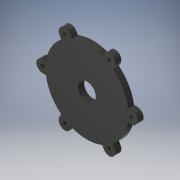
# Autodesk Inventor part: TA01
Saved by Autodesk Inventor 2017 (Build 210142000, 142)
## iProperties
Created: 2018-10-09
Part Number: TA01
Material: ABS Plastic
Document SubType Name: Modeling
Designer: Zach
Density: 1.06 g/cm^3
Appearance: Smooth - Black
Author: Zach
Autodesk Inventor part; units mm, degrees
ref_plane "YZ Plane" through (0, 0, 0) normal (1, 0, 0) x (0, 1, 0)
ref_plane "XZ Plane" through (0, 0, 0) normal (0, 1, 0) x (-1, 0, 0)
ref_plane "XY Plane" through (0, 0, 0) normal (0, 0, 1) x (1, 0, 0)
sketch "Sketch1" plane through (0, 0, 0) normal (0, 0, 1) x (1, 0, 0)
  circle A0 centre (0, 0) radius 15
  circle A1 centre (0, 0) radius 68.75
  circle A2 centre (-50, 0) radius 3
  circle A3 centre (-25, -43.3013) radius 3
  circle A4 centre (25, -43.3013) radius 3
  circle A5 centre (50, 0) radius 3
  circle A6 centre (25, 43.3013) radius 3
  circle A7 centre (-25, 43.3013) radius 3
  dimension "d0" = 30
  dimension "d1" = 137.5
  dimension "d2" = 6
  dimension "d6" = 360
  dimension "d15" = 50
  constraints: 8 centre point, 2 coincident, 1 horizontal alignment, 13 other
  measures "d0" diameter of A0
  measures "d1" diameter of A1
  measures "d2" diameter of A2
  measures "d15" distance of point (0, 0) A2.centre
extrude "Extrusion1" add sketch "Sketch1" along normal blind 10 contours A1 | A2 | A3 | A4 | A5 | A6 | A7
sketch "Sketch5" plane through (0, 0, 0) normal (0, 0, -1) x (-1, 0, 0)
  circle A0 centre (74, 0) radius 10
  line L0 (74, 10) -> (68.0188, 10)
  line L1 (74, -10) -> (68.0188, -10)
  line L2 (68.0188, 10) -> (68.0188, -10)
  circle A1 centre (74, 0) radius 3
  circle A2 centre (0, 0) radius 68.75 construction
  line L3 (74, 0) -> (0, 0) construction
  circle A3 centre (50.5575, 0) radius 3 construction
  circle A4 centre (37, 64.0859) radius 10
  line L4 (28.3397, 69.0859) -> (25.3492, 63.906)
  line L5 (45.6603, 59.0859) -> (42.6697, 53.906)
  line L6 (25.3492, 63.906) -> (42.6697, 53.906)
  circle A5 centre (37, 64.0859) radius 3
  circle A6 centre (-37, 64.0859) radius 10
  line L7 (-45.6603, 59.0859) -> (-42.6697, 53.906)
  line L8 (-28.3397, 69.0859) -> (-25.3492, 63.906)
  line L9 (-42.6697, 53.906) -> (-25.3492, 63.906)
  circle A7 centre (-37, 64.0859) radius 3
  circle A8 centre (-74, 0) radius 10
  line L10 (-74, -10) -> (-68.0188, -10)
  line L11 (-74, 10) -> (-68.0188, 10)
  line L12 (-68.0188, -10) -> (-68.0188, 10)
  circle A9 centre (-74, 0) radius 3
  circle A10 centre (-37, -64.0859) radius 10
  line L13 (-28.3397, -69.0859) -> (-25.3492, -63.906)
  line L14 (-45.6603, -59.0859) -> (-42.6697, -53.906)
  line L15 (-25.3492, -63.906) -> (-42.6697, -53.906)
  circle A11 centre (-37, -64.0859) radius 3
  circle A12 centre (37, -64.0859) radius 10
  line L16 (45.6603, -59.0859) -> (42.6697, -53.906)
  line L17 (28.3397, -69.0859) -> (25.3492, -63.906)
  line L18 (42.6697, -53.906) -> (25.3492, -63.906)
  circle A13 centre (37, -64.0859) radius 3
  circle A14 centre (0, 0) radius 15 projected
  circle A15 centre (0, 0) radius 68.75 projected
  dimension "d24" = 20
  dimension "d25" = 6
  dimension "d26" = 74
  dimension "d29" = 360
  constraints: 38 end point, 14 centre point, 14 point on circle, 8 coincident, 2 parallel, 2 tangent, 1 horizontal alignment, 1 point on line, 69 other
  measures "d24" diameter of A0
  measures "d25" diameter of A1
  measures "d26" distance of L3.start L3.end
extrude "Extrusion4" add sketch "Sketch5" against normal blind 10 contours A0 A15 | A0 A15 L0 | L1 A15 A0 | A15 A0 L2 | A0 L2 A15 | A15 L2 A0 | L2 A0 | A15 A4 L5 | L6 A4 A15 | A15 A12 L18 | L16 A12 A15 | A4 A15 | L6 A4 A15 | A4 L6 | A12 A15 | L18 A12 | A12 A15 L18 | L6 A15 A4 | A15 L4 A4 | A12 A15 L18 | A12 L17 A15 | A15 A6 L8 | L9 A6 A15 | A15 A10 L15 | L13 A10 A15 | A6 A15 | L9 A6 A15 | A6 L9 | A10 A15 | L15 A10 | A10 A15 L15 | A6 A15 L7 | L9 A15 A6 | L14 A15 A10 | A10 A15 L15 | A15 A8 L11 | L12 A8 A15 | A15 A8 L12 | L10 A8 A15 | A8 A15 | L12 A8 A15 | A8 L12
body "Solid1"
